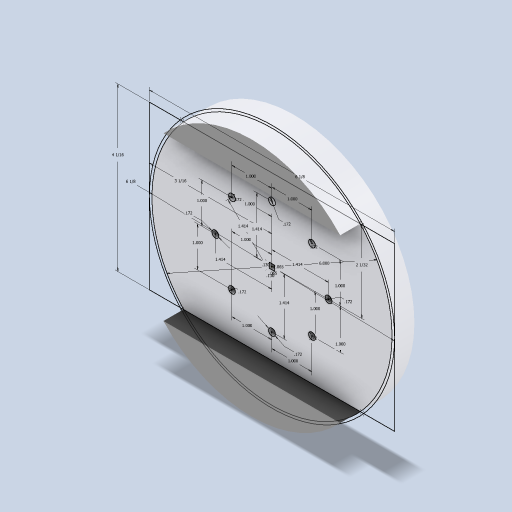
# Autodesk Inventor part: rocker wheel
Saved by Autodesk Inventor 2023 (Build 270158000, 158)
## iProperties
Created: 2022-11-04
Part Number: rocker wheel
Material: Generic
Document SubType Name: Modeling
Designer: Nathan
Density: 1 g/cm^3
Appearance: No Tint
Author: Nathan
Autodesk Inventor part; units mm, degrees
ref_plane "YZ Plane" through (0, 0, 0) normal (1, 0, 0) x (0, 1, 0)
ref_plane "XZ Plane" through (0, 0, 0) normal (0, 1, 0) x (-1, 0, 0)
ref_plane "XY Plane" through (0, 0, 0) normal (0, 0, 1) x (1, 0, 0)
sketch "Sketch1" plane through (0, 0, 0) normal (0, 0, 1) x (1, 0, 0)
  circle A0 centre (0, 0) radius 76.2
  circle A1 centre (-25.4, 25.4) radius 2.1844
  circle A2 centre (25.4, 25.4109) radius 2.1844
  circle A3 centre (-25.4, -25.4) radius 2.1844
  circle A4 centre (25.4, -25.4) radius 2.1844
  circle A5 centre (0.0108, 35.9156) radius 2.1844
  circle A6 centre (35.9264, 0) radius 2.1844
  circle A7 centre (-35.9156, 0) radius 2.1844
  circle A8 centre (0, -35.9264) radius 2.1844
  circle A9 centre (0, 0) radius 77.7875
  line L0 (77.7875, 51.5938) -> (-77.7875, 51.5937)
  line L1 (-77.7875, 51.5937) -> (-77.7875, -51.5938)
  line L2 (-77.7875, -51.5938) -> (77.7875, -51.5937)
  line L3 (77.7875, -51.5937) -> (77.7875, 51.5938)
  line L4 (1.651, 1.651) -> (-1.651, 1.651)
  line L5 (-1.651, 1.651) -> (-1.651, -1.651)
  line L6 (-1.651, -1.651) -> (1.651, -1.651)
  line L7 (1.651, -1.651) -> (1.651, 1.651)
  point P0 (56.0761, -51.5937)
  point P1 (-56.0761, -51.5938)
  point P2 (-56.0761, 51.5938)
  point P3 (56.0761, 51.5938)
  point P4 (-58.2149, 51.5938)
  point P5 (-56.0761, 51.5938)
  point P6 (56.0761, 51.5938)
  point P7 (58.2149, 51.5938)
  point P8 (56.0761, -51.5937)
  point P9 (58.2149, -51.5937)
  point P10 (-58.2149, -51.5938)
  point P11 (-56.0761, -51.5938)
  dimension "d0" = 152.4
  dimension "d5" = 4.3688
  dimension "d6" = 4.3688
  dimension "d7" = 4.3688
  dimension "d8" = 4.3688
  dimension "d15" = 4.3688
  dimension "d16" = 4.3688
  dimension "d17" = 4.3688
  dimension "d18" = 4.3688
  dimension "d19" = 155.575
  dimension "d20" = 35.9156
  dimension "d21" = 35.921
  dimension "d22" = 25.3892
  dimension "d23" = 25.4108
  dimension "d24" = 25.4
  dimension "d25" = 25.4
  dimension "d26" = 25.4
  dimension "d27" = 25.4
  dimension "d28" = 25.4
  dimension "d29" = 25.4108
  dimension "d30" = 25.4
  dimension "d31" = 35.9156
  dimension "d32" = 25.4
  dimension "d33" = 35.9265
  dimension "d34" = 25.4
  dimension "d35" = 35.9265
  dimension "d38" = 155.575
  dimension "d39" = 103.1875
  dimension "d40" = 51.5938
  dimension "d41" = 77.7875
  dimension "d47" = 3.302
  dimension "d48" = 3.302
  dimension "d49" = 1.651
  dimension "d50" = 1.651
  constraints: 16 end point, 10 centre point, 8 point on circle, 8 point on line, 4 parallel, 2 coincident, 2 horizontal, 2 perpendicular
  measures "d0" diameter of A0
  measures "d5" diameter of A1
  measures "d6" diameter of A2
  measures "d7" diameter of A3
  measures "d8" diameter of A4
  measures "d15" diameter of A5
  measures "d16" diameter of A6
  measures "d17" diameter of A7
  measures "d18" diameter of A8
  measures "d19" diameter of A9
  measures "d20" distance of point (0, 0) A5.centre
  measures "d21" distance of point (0, 0) A1.centre
  measures "d22" horizontal distance of A2.centre A5.centre
  measures "d23" vertical distance of A6.centre A2.centre
  measures "d24" vertical distance of A4.centre A6.centre
  measures "d25" horizontal distance of A8.centre A4.centre
  measures "d26" horizontal distance of A8.centre A3.centre
  measures "d27" vertical distance of A7.centre A3.centre
  measures "d28" vertical distance of A1.centre A7.centre
  measures "d29" horizontal distance of A5.centre A1.centre
  measures "d30" horizontal distance of point (0, 0) A1.centre
  measures "d31" distance of A0.centre A7.centre
  measures "d32" horizontal distance of A9.centre A3.centre
  measures "d33" distance of point (0, 0) A8.centre
  measures "d34" horizontal distance of point (0, 0) A4.centre
  measures "d35" distance of A0.centre A6.centre
  measures "d38" distance of L0.start L0.end
  measures "d39" distance of L0.end L1.end
  measures "d40" distance from line of point (0, 0) L0
  measures "d41" distance from line of L1 point (0, 0)
  measures "d47" distance of L4.end L5.end
  measures "d48" distance of L5.end L6.end
  measures "d49" distance from line of L4 point (0, 0)
  measures "d50" distance from line of L7 A9.centre
extrude "Extrusion6" add sketch "Sketch1" against normal blind 14.2875 contours A0 L2 L0 | L0 A0 | A0 L2
extrude "Extrusion8" add sketch "Sketch1" along normal blind 12.7 contours L0 A0 | A0 L2
body "Solid4"
